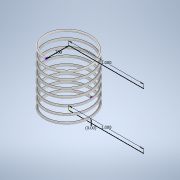
# Autodesk Inventor part: filiment
Saved by Autodesk Inventor 2020 (Build 240168000, 168)
## iProperties
Created: 2019-06-18
Part Number: filiment
Material: Generic
Document SubType Name: Modeling
Designer: ColinP
Density: 1 g/cm^3
Appearance: Default
Author: ColinP
Autodesk Inventor part; units mm, degrees
ref_plane "YZ Plane" through (0, 0, 0) normal (1, 0, 0) x (0, 1, 0)
ref_plane "XZ Plane" through (0, 0, 0) normal (0, 1, 0) x (-1, 0, 0)
ref_plane "XY Plane" through (0, 0, 0) normal (0, 0, 1) x (1, 0, 0)
sketch "Sketch1" plane through (0, 0, 0) normal (0, 1, 0) x (-1, 0, 0)
  line L0 (0, 0) -> (0, 7.62)
  dimension "d1" = 7.62
  constraints: 2 end point, 1 vertical
  measures "d1" distance of L0.start L0.end
sketch "Sketch3" plane through (0, 0, 0) normal (1, 0, 0) x (0, 1, 0)
  circle A0 centre (0, 7.6145) radius 0.381
  point P0 (0, 0)
  dimension "d3" = 0.762
  constraints: 1 centre point
  measures "d3" diameter of A0
sketch "Sketch2" plane through (0, 0, 0) normal (1, 0, 0) x (0, 1, 0)
  line L0 (0.8114, 0) -> (-0.5168, 0)
  point P0 (0, 0)
  constraints: 2 end point, 1 horizontal
coil "Coil1" sketch "Sketch3" operation add axis through (0, 0.8114, 0) along (0, -1, 0) pitch 2.54 turns 7.5 hand right
sketch "Sketch4" plane through (0, 0, 0) normal (1, 0, 0) x (0, 1, 0)
  point P0 (0, 0)
sketch "Sketch5" plane through (0, 0, 0) normal (0, 0, 1) x (1, 0, 0)
  line L0 (-11.0101, -4.6555) -> (-11.0101, -5.4276)
  point P0 (0, 0)
  constraints: 2 end point, 1 vertical
sketch "Sketch6" plane through (0, 0, 0) normal (0, 0, 1) x (1, 0, 0)
  line L0 (0, 0) -> (25.4, 0)
  line L1 (0, -19.431) -> (0, -18.669) projected
  line L2 (0, -19.05) -> (25.4, -19.05)
  line L3 (0, -19.05) -> (25.4, -19.05) construction
  dimension "d12" = 25.4
  dimension "d13" = 25.4
  dimension "d14" = 0
  constraints: 6 end point, 3 horizontal, 1 collinear, 1 midpoint
  measures "d12" distance of L0.start L0.end
  measures "d13" distance of L2.start L2.end
  measures "d14" distance between parallel lines of L2 L3
sketch "Sketch7" plane through (0, 0, 0) normal (1, 0, 0) x (0, 1, 0)
  circle A0 centre (0, 7.6145) radius 0.381 projected
  circle A1 centre (0, 7.6145) radius 0.381
  circle A2 centre (-19.05, -7.6145) radius 0.381 projected
  circle A3 centre (-19.05, -7.6145) radius 0.381
  point P0 (0, 0)
  point P1 (0.381, 7.6145)
  point P2 (-18.669, -7.6145)
  constraints: 2 centre point, 2 coincident, 2 horizontal alignment
sketch "Sketch8" plane through (0, 0, 0) normal (0, 1, 0) x (-1, 0, 0)
  point P0 (0, 0)
body "Solid1"
